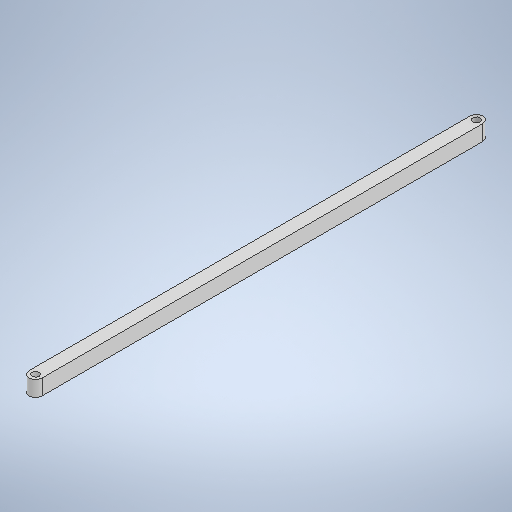
# Autodesk Inventor part: scrambler_spider_support2
Saved by Autodesk Inventor 2025.2 (Build 292293000, 293)
## iProperties
Created: 2025-10-14
Part Number: scrambler_spider_support2
Material: Generic
Document SubType Name: Modeling
Designer: pascu
Density: 1 g/cm^3
Appearance: Default
Author: pascu
Autodesk Inventor part; units mm, degrees
ref_plane "YZ Plane" through (0, 0, 0) normal (1, 0, 0) x (0, 1, 0)
ref_plane "XZ Plane" through (0, 0, 0) normal (0, 1, 0) x (-1, 0, 0)
ref_plane "XY Plane" through (0, 0, 0) normal (0, 0, 1) x (1, 0, 0)
sketch "Sketch1" plane through (0, 0, 0) normal (0, 1, 0) x (-1, 0, 0)
  line L0 (-3.175, 0) -> (-3.175, -108.2294)
  line L1 (0, -108.2294) -> (0, 0)
  arc A0 (0, 0) -> (-3.175, 0) centre (-1.5875, 0) ccw
  arc A1 (-3.175, -108.2294) -> (0, -108.2294) centre (-1.5875, -108.2294) ccw
  dimension "d0" = 3.175
  dimension "d1" = 108.2294
  constraints: 4 end point, 4 point on circle, 2 centre point, 1 parallel
  measures "d0" distance of L1.start L0.end
  measures "d1" distance of L0.end L0.start
extrude "Extrusion1" add sketch "Sketch1" along normal blind 3.81
sketch "Sketch2" plane through (0, 3.81, 0) normal (0, 1, 0) x (1, 0, 0)
  arc A0 (0, 0) -> (3.175, 0) centre (1.5875, 0) ccw projected
  circle A1 centre (1.5875, 0) radius 0.889
  arc A2 (3.175, 108.2294) -> (0, 108.2294) centre (1.5875, 108.2294) ccw projected
  circle A3 centre (1.5875, 108.2294) radius 0.889
  dimension "d4" = 1.778
  constraints: 2 centre point, 2 coincident
  measures "d4" diameter of A1
extrude "Extrusion2" cut sketch "Sketch2" against normal blind 3.81
body "Solid1"
